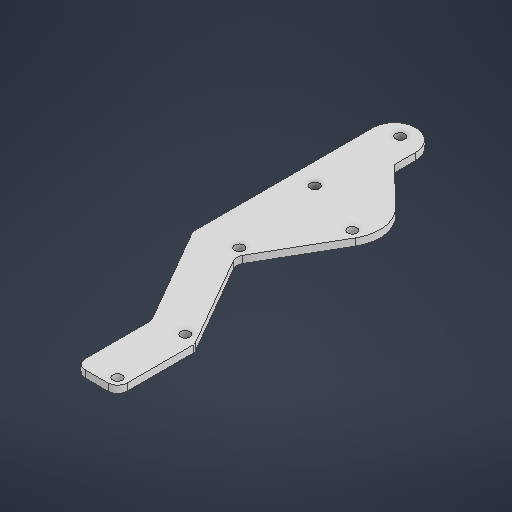
# Autodesk Inventor part: ClawGrabPlate
Saved by Autodesk Inventor 2025 (Build 290162000, 162)
## iProperties
Created: 2024-05-20
Part Number: ClawGrabPlate
Material: Generic
Document SubType Name: Modeling
Designer: avsar
Density: 1 g/cm^3
Appearance: Default
Author: avsar
Autodesk Inventor part; units mm, degrees
ref_plane "YZ Plane" through (0, 0, 0) normal (1, 0, 0) x (0, 1, 0)
ref_plane "XZ Plane" through (0, 0, 0) normal (0, 1, 0) x (-1, 0, 0)
ref_plane "XY Plane" through (0, 0, 0) normal (0, 0, 1) x (1, 0, 0)
sketch "Sketch1" plane through (0, 0, 0) normal (0, 1, 0) x (-1, 0, 0)
  line L0 (9, 30.5) -> (-9, 30.5) construction
  line L1 (-9, 30.5) -> (-9, -12.5) construction
  line L2 (-9, -30.5) -> (9, -30.5)
  line L3 (9, 30.5) -> (-9, -30.5) construction
  line L4 (-9, 30.5) -> (9, -30.5) construction
  circle A0 centre (0, -24) radius 2
  circle A1 centre (0, 12) radius 2
  line L5 (9, 30.5) -> (-9, 30.5) construction
  line L6 (-33.8261, 11.5) -> (-15.8261, 11.5) construction
  line L7 (-33.8261, 11.5) -> (-9, 54.5)
  line L8 (-15.8261, 11.5) -> (14.1464, 63.4139) construction
  line L9 (-9, 54.5) -> (-33.8261, 97.5)
  line L10 (9, 54.5) -> (-15.8261, 97.5)
  line L11 (-33.8261, 97.5) -> (-15.8261, 97.5)
  line L12 (-15.8261, 11.5) -> (9, 11.5) construction
  line L13 (-9, -12.5) -> (-33.8261, 11.5)
  line L14 (-9, -12.5) -> (-9, -30.5)
  line L15 (9, -30.5) -> (9, 11.5)
  line L16 (9, 11.5) -> (9, 54.5)
  point P0 (0, 0)
  dimension "d0" = 18
  dimension "d1" = 61
  dimension "d2" = 4
  dimension "d3" = 24
  dimension "d4" = 4
  dimension "d5" = 36
  dimension "d8" = 18
  dimension "d9" = 43
  dimension "d10" = 60
  dimension "d11" = 120
  dimension "d14" = 18
  dimension "d15" = 24
  constraints: 34 end point, 5 parallel, 3 horizontal, 2 centre point, 2 midpoint, 2 perpendicular, 2 vertical alignment, 1 collinear, 1 equal length, 1 horizontal alignment, 1 point on line, 1 vertical
  measures "d0" distance of L2.end L2.start
  measures "d1" distance of L2.start L0.end
  measures "d2" diameter of A0
  measures "d3" distance of point (0, 0) A0.centre
  measures "d4" diameter of A1
  measures "d5" distance of A0.centre A1.centre
  measures "d8" distance of L6.start L6.end
  measures "d9" vertical distance of L7.end L6.end
  measures "d10" angle of L6 L7
  measures "d11" angle of L9 L7
  measures "d14" distance of L2.start L1.end
  measures "d15" vertical distance of L1.end L6.start
extrude "Extrusion1" add sketch "Sketch1" along normal blind 3
fillet "Fillet1" radius 16 1 edges at (33.8261, 1.5, 11.5)
fillet "Fillet2" radius 4 1 edges at (9, 1.5, 54.5)
fillet "Fillet3" radius 2 1 edges at (33.8261, 1.5, 97.5)
fillet "Fillet4" radius 4 2 edges at (15.8261, 1.5, 97.5) (-9, 1.5, 54.5)
fillet "Fillet5" radius 9 2 edges at (9, 1.5, -30.5) (-9, 1.5, -30.5)
sketch "Sketch2" plane through (0, 3, 0) normal (0, 1, 0) x (1, 0, 0)
  arc A0 (9, 21.5) -> (-9, 21.5) centre (0, 21.5) ccw construction
  line L0 (-9, 21.5) -> (-9, -53.4282) construction
  arc A1 (-9, -53.4282) -> (-8.4641, -55.4282) centre (-5, -53.4282) ccw construction
  line L1 (-8.4641, -55.4282) -> (14.6714, -95.5) construction
  arc A2 (14.6714, -95.5) -> (18.1355, -97.5) centre (18.1355, -93.5) ccw construction
  line L2 (18.1355, -97.5) -> (30.362, -97.5) construction
  arc A3 (30.362, -97.5) -> (32.094, -94.5) centre (30.362, -95.5) ccw construction
  line L3 (32.094, -94.5) -> (10.1547, -56.5) construction
  arc A4 (10.1547, -52.5) -> (10.1547, -56.5) centre (13.6188, -54.5) ccw construction
  line L4 (10.1547, -52.5) -> (27.5792, -22.3198) construction
  arc A5 (27.5792, -22.3198) -> (24.8435, -2.8164) centre (13.7228, -14.3198) ccw construction
  line L5 (24.8435, -2.8164) -> (9, 12.5) construction
  line L6 (9, 12.5) -> (9, 21.5) construction
  circle A6 centre (0, -12) radius 2 construction
  circle A7 centre (0, 24) radius 2 construction
  line L7 (5.6099, 10.2137) -> (22.0634, -5.6922) construction
  arc A8 (24.1151, -20.3198) -> (22.0634, -5.6922) centre (13.7228, -14.3198) ccw construction
  line L8 (24.1151, -20.3198) -> (6.6906, -50.5) construction
  arc A9 (6.6906, -50.5) -> (6.6906, -58.5) centre (13.6188, -54.5) ccw construction
  line L9 (6.6906, -58.5) -> (26.8979, -93.5) construction
  line L10 (26.8979, -93.5) -> (18.1355, -93.5)
  line L11 (18.1355, -93.5) -> (-5, -53.4282)
  line L12 (-5, -53.4282) -> (-5, 21.5)
  arc A10 (5, 21.5) -> (-5, 21.5) centre (0, 21.5) ccw
  line L13 (5, 21.5) -> (5, 11.6517) construction
  circle A11 centre (5, 10.8034) radius 2
  arc A12 (5, 11.6517) -> (5.6099, 10.2137) centre (7, 11.6517) ccw construction
  circle A13 centre (22.0634, -5.6922) radius 2
  circle A14 centre (24.1151, -20.3198) radius 2
  circle A15 centre (6.6906, -50.5) radius 2
  circle A16 centre (26.8979, -93.5) radius 2
  point P0 (0, 0)
  dimension "d22" = 4
  dimension "d23" = 4
  dimension "d26" = 2
  dimension "d27" = 4
  dimension "d28" = 4
  dimension "d29" = 4
  dimension "d30" = 4
  constraints: 14 end point, 9 centre point, 9 point on circle, 4 coincident, 2 point on line, 2 tangent, 9 other
  measures "d22" distance between parallel lines of L5 L7
  measures "d23" diameter of A11
  measures "d26" radius of A12
  measures "d27" diameter of A13
  measures "d28" diameter of A14
  measures "d29" diameter of A15
  measures "d30" diameter of A16
sketch "Sketch3" plane through (0, 3, 0) normal (0, 1, 0) x (1, 0, 0)
  arc A0 (30.362, -97.5) -> (32.094, -94.5) centre (30.362, -95.5) ccw projected
  line L0 (32.362, -95.5) -> (32.362, -127.5)
  line L1 (32.362, -127.5) -> (14.6714, -127.5)
  arc A1 (14.6714, -95.5) -> (18.1355, -97.5) centre (18.1355, -93.5) ccw projected
  line L2 (14.6714, -127.5) -> (14.6714, -95.5)
  line L3 (18.1355, -97.5) -> (30.362, -97.5) projected
  point P0 (0, 0)
  dimension "d31" = 32
  constraints: 6 end point, 2 vertical, 1 perpendicular, 1 point on circle, 1 tangent
  measures "d31" distance of L0.start L0.end
extrude "Extrusion3" add sketch "Sketch3" against normal up to surface (3 mm away)
fillet "Fillet6" radius 4 3 edges at (14.6714, 1.5, 95.5) (14.6714, 1.5, 127.5) (32.362, 1.5, 127.5)
extrude "Extrusion2" cut sketch "Sketch2" against normal through all contours A14 | A15 | A16
sketch "Sketch4" plane through (0, 3, 0) normal (0, 1, 0) x (1, 0, 0)
  circle A0 centre (28.362, -123.5) radius 2
  line L0 (32.362, -123.5) -> (32.362, -95.5) projected
  line L1 (18.6714, -127.5) -> (28.362, -127.5) projected
  point P0 (0, 0)
  dimension "d35" = 4
  dimension "d36" = 4
  dimension "d37" = 4
  constraints: 1 centre point
  measures "d35" diameter of A0
  measures "d36" distance from line of L0 A0.centre
  measures "d37" distance from line of L1 A0.centre
extrude "Extrusion4" cut sketch "Sketch4" against normal through all
equation "\"d11\" = 2 * d10"
body "Solid1"
